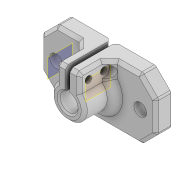
# Autodesk Inventor part: Joint_Mount
Saved by Autodesk Inventor 2020 (Build 240168000, 168)
## iProperties
Created: 2022-01-08
Part Number: Joint_Mount
Material: 一般
Document SubType Name: Modeling
Designer: ken113
Density: 1 g/cm^3
Appearance: 既定
Author: ken113
Autodesk Inventor part; units mm, degrees
ref_plane "YZ Plane" through (0, 0, 0) normal (1, 0, 0) x (0, 1, 0)
ref_plane "XZ Plane" through (0, 0, 0) normal (0, 1, 0) x (-1, 0, 0)
ref_plane "XY Plane" through (0, 0, 0) normal (0, 0, 1) x (1, 0, 0)
sketch "スケッチ1" plane through (0, 0, 0) normal (0, 0, 1) x (1, 0, 0)
  line L0 (37.5, -20) -> (-37.5, -20)
  line L1 (-37.5, -20) -> (-37.5, 20)
  line L2 (-37.5, 20) -> (37.5, 20)
  line L3 (37.5, 20) -> (37.5, -20)
  line L4 (37.5, -20) -> (-37.5, 20) construction
  line L5 (-37.5, -20) -> (37.5, 20) construction
  point P0 (0, 0)
  dimension "d0" = 40
  dimension "d1" = 75
  constraints: 12 end point, 2 midpoint, 2 parallel, 1 horizontal, 1 perpendicular
  measures "d0" distance of L0.end L1.end
  measures "d1" distance of L1.end L2.end
extrude "押し出し1" add sketch "スケッチ1" along normal blind 10
sketch "スケッチ2" plane through (0, 0, 10) normal (0, 0, 1) x (1, 0, 0)
  circle A0 centre (0, 0) radius 5.9
  dimension "d4" = 11.8
  constraints: 1 centre point, 1 coincident
  measures "d4" diameter of A0
extrude "押し出し2" cut sketch "スケッチ2" against normal blind 10
sketch "スケッチ3" plane through (0, 0, 10) normal (0, 0, 1) x (1, 0, 0)
  circle A0 centre (0, 0) radius 5.9
  circle A1 centre (0, 0) radius 10.9
  line L0 (-1.5, 0) -> (1.5, 0)
  line L1 (1.5, 0) -> (1.5, 13.624508)
  line L2 (1.5, 13.624508) -> (-1.5, 13.624508)
  line L3 (-1.5, 13.624508) -> (-1.5, 0)
  point P0 (-1.5, 5.706137)
  point P1 (-1.5, 10.796296)
  point P2 (1.5, 10.796296)
  point P3 (1.5, 5.706137)
  dimension "d7" = 5
  dimension "d8" = 3
  dimension "d9" = 1.5
  constraints: 8 end point, 2 centre point, 2 parallel, 1 coincident, 1 horizontal, 1 perpendicular
  measures "d7" radial gap between concentric circles of A0 A1
  measures "d8" distance of L1.end L2.end
  measures "d9" distance from line of point (0, 0) L3
extrude "押し出し3" add sketch "スケッチ3" along normal blind 20 contours A0 L1 A1 L3 picked at (9.128542, -0.866316)
sketch "スケッチ4" plane through (0, 0, 10) normal (0, 0, 1) x (1, 0, 0)
  line L0 (-1.5, 10.796296) -> (-1.5, 5.706137)
  arc A0 (1.5, 5.706137) -> (-1.5, 5.706137) centre (0, 0) ccw
  line L1 (1.5, 5.706137) -> (1.5, 10.796296)
  arc A1 (-1.5, 10.796296) -> (1.5, 10.796296) centre (0, 0) ccw
  line L2 (-37.5, -20) -> (37.5, -20)
  line L3 (37.5, -20) -> (37.5, 20)
  line L4 (37.5, 20) -> (-37.5, 20)
  line L5 (-37.5, 20) -> (-37.5, -20)
  line L6 (37.5, 20) -> (-37.5, 20)
  line L7 (1.5, 5.706137) -> (-1.5, 5.706137)
  line L8 (-1.5, 5.706137) -> (-1.5, 20)
  line L9 (-1.5, 20) -> (1.5, 20)
  line L10 (1.5, 20) -> (1.5, 5.706137)
  constraints: 8 end point, 2 parallel, 1 horizontal, 1 perpendicular, 1 point on line, 1 vertical alignment
extrude "押し出し4" cut sketch "スケッチ4" against normal blind 20 contours L8 L4 L10 L1 A0 L0
sketch "スケッチ5" plane through (0, 0, 30) normal (0, 0, 1) x (1, 0, 0)
  arc A0 (-1.5, 5.706137) -> (1.5, 5.706137) centre (0, 0) ccw
  line L0 (-1.5, 5.706137) -> (-1.5, 10.796296)
  arc A1 (-1.5, 10.796296) -> (1.5, 10.796296) centre (0, 0) ccw
  line L1 (1.5, 10.796296) -> (1.5, 5.706137)
  line L2 (-1.5, 10.796296) -> (-1.5, 20)
  line L3 (-1.5, 20) -> (-37.5, 20)
  line L4 (-37.5, 20) -> (-37.5, -20)
  line L5 (-37.5, -20) -> (37.5, -20)
  line L6 (37.5, -20) -> (37.5, 20)
  line L7 (37.5, 20) -> (1.5, 20)
  line L8 (1.5, 20) -> (1.5, 10.796296)
  arc A2 (-1.5, 10.796296) -> (1.5, 10.796296) centre (0, 0) ccw
  line L9 (7.5, 1.842007) -> (-7.5, 1.842007)
  line L10 (-7.5, 1.842007) -> (-7.5, 20)
  line L11 (-7.5, 20) -> (7.5, 20)
  line L12 (7.5, 20) -> (7.5, 1.842007)
  point P0 (-1.5, 20)
  point P1 (-7.5, 7.909488)
  point P2 (-1.5, 10.796296)
  point P3 (7.5, 7.909488)
  point P4 (1.5, 20)
  point P5 (1.5, 10.796296)
  dimension "d14" = 6
  dimension "d15" = 6
  constraints: 8 end point, 2 parallel, 1 horizontal, 1 horizontal alignment, 1 perpendicular
  measures "d14" distance between parallel lines of L12 L8
  measures "d15" distance between parallel lines of L10 L2
extrude "押し出し5" add sketch "スケッチ5" against normal up to surface (20 mm away) contours A1 L10 L3 L2 | A1 L8 L7 L12
chamfer "面取り1" distance 5 angle 45 3 edges at (7.5, 13.9547, 10) (0, -10.9, 10) (-7.5, 13.9547, 10)
chamfer "面取り2" distance 2 angle 45 2 edges at (4.5, 20, 30) (-4.5, 20, 30)
chamfer "面取り3" distance 10 angle 45 4 edges at (-37.5, 20, 5) (-37.5, -20, 5) (37.5, 20, 5) (37.5, -20, 5)
chamfer "面取り4" distance 1 angle 45 1 edges at (0, -5.9, 30)
ref_plane "作業平面1" through (12.5, 7.909488, 15) normal (1, 0, 0) x (0, 0, -1)
sketch "スケッチ6" plane through (12.5, 7.909488, 15) normal (1, 0, 0) x (0, 0, -1)
  line L0 (5, 1.917007) -> (5, 12.090512)
  line L1 (5, 12.090512) -> (0, 12.090512)
  line L2 (0, 12.090512) -> (0, 0)
  line L3 (-15, 10.090512) -> (-13, 12.090512)
  line L4 (-15, 0) -> (-15, 10.090512)
  line L5 (0, 0) -> (-15, 0)
  line L6 (0, 12.090512) -> (0, 0)
  line L7 (-13, 12.090512) -> (0, 12.090512)
  point P0 (15, -7.909488)
  point P1 (-9, 6.090512)
  point P2 (1, 6.090512)
  dimension "d32" = 6
  dimension "d33" = 6
  dimension "d34" = 6
  dimension "d35" = 16
  constraints: 1 other
  measures "d32" distance from line of point (-9, 6.091) L7
  measures "d33" distance from line of L7 point (1, 6.091)
  measures "d34" distance from line of point (-9, 6.091) L4
  measures "d35" distance from line of point (1, 6.091) L4
hole "穴1" at (12.5, 14, 24) at (12.5, 14, 14) direction (-1, 0, 0) diameter 4.3 end through all counterbore diameter 8 counterbore depth 5
ref_plane "作業平面2" through (-12.5, 7.909488, 15) normal (-1, 0, 0) x (0, 0, 1)
sketch "スケッチ7" plane through (-12.5, 7.909488, 15) normal (-1, 0, 0) x (0, 0, 1)
  arc A0 (0, 4.187225) -> (0, 7.993799) centre (-1, 6.090512) ccw
  line L0 (0, 0) -> (0, 4.187225)
  line L1 (15, 0) -> (0, 0)
  line L2 (15, 10.090512) -> (15, 0)
  line L3 (13, 12.090512) -> (15, 10.090512)
  line L4 (13, 12.090512) -> (0, 12.090512)
  line L5 (0, 7.993799) -> (0, 12.090512)
  circle A1 centre (9, 6.090512) radius 2.15
  arc A2 (0, 7.993799) -> (0, 4.187225) centre (-1, 6.090512) ccw
  circle A3 centre (9, 6.090512) radius 2.15
  line L6 (4.843078, 6.090512) -> (6.921539, 9.690512)
  line L7 (6.921539, 9.690512) -> (11.078461, 9.690512)
  line L8 (11.078461, 9.690512) -> (13.156922, 6.090512)
  line L9 (13.156922, 6.090512) -> (11.078461, 2.490512)
  line L10 (11.078461, 2.490512) -> (6.921539, 2.490512)
  line L11 (6.921539, 2.490512) -> (4.843078, 6.090512)
  line L12 (3.156922, 6.090512) -> (1.078461, 2.490512)
  line L13 (1.078461, 2.490512) -> (-3.078461, 2.490512)
  line L14 (-3.078461, 2.490512) -> (-5.156922, 6.090512)
  line L15 (-5.156922, 6.090512) -> (-3.078461, 9.690512)
  line L16 (-3.078461, 9.690512) -> (1.078461, 9.690512)
  line L17 (1.078461, 9.690512) -> (3.156922, 6.090512)
  point P0 (-15, -7.909488)
  dimension "d44" = 7.2
  dimension "d45" = 7.2
  constraints: 24 end point, 2 coincident, 1 horizontal alignment, 26 other
  measures "d44" distance between parallel lines of L10 L7
  measures "d45" distance between parallel lines of L13 L16
extrude "押し出し6" cut sketch "スケッチ7" against normal blind 7 contours A0 L5 L16 L17 L12 L13 L0 | L0 L13 L14 L15 L16 L5 A2 | L6 L7 L8 L9 L10 L11
chamfer "面取り5" distance 2 angle 45 2 edges at (1.5, 12.8531, 0) (-1.5, 12.8531, 0)
sketch "スケッチ8" plane through (0, 0, 10) normal (0, 0, 1) x (1, 0, 0)
  line L0 (37.5, -10) -> (27.5, -20)
  line L1 (37.5, -10) -> (37.5, 10)
  line L2 (27.5, 20) -> (37.5, 10)
  line L3 (27.5, 20) -> (12.5, 20)
  line L4 (12.5, 9.826495) -> (12.5, 14)
  arc A0 (-12.5, 9.826495) -> (12.5, 9.826495) centre (0, 0) ccw
  line L5 (-12.5, 20) -> (-12.5, 14.271797)
  line L6 (-12.5, 20) -> (-27.5, 20)
  line L7 (-37.5, 10) -> (-27.5, 20)
  line L8 (-37.5, 10) -> (-37.5, -10)
  line L9 (-27.5, -20) -> (-37.5, -10)
  line L10 (-27.5, -20) -> (27.5, -20)
  line L11 (12.5, 14) -> (12.5, 20)
  line L12 (-12.5, 13.728203) -> (-12.5, 9.826495)
  line L13 (-12.5, 14.271797) -> (-12.5, 13.728203)
  point P0 (27.5, 0)
  point P1 (-27.5, 0)
  dimension "d51" = 10
  dimension "d52" = 10
  measures "d51" distance from line of point (27.5, 0) L1
  measures "d52" distance from line of L8 point (-27.5, 0)
hole "穴2" at (27.5, 0, 10) at (-27.5, 0, 10) direction (0, 0, -1) diameter 8.3 end through all
fillet "フィレット1" radius 2 8 edges at (27.5, -20, 5) (37.5, -10, 5) (37.5, 10, 5) (27.5, 20, 5) (-27.5, 20, 5) (-37.5, 10, 5) (-37.5, -10, 5) (-27.5, -20, 5)
chamfer "面取り6" distance 2 angle 45 26 edges at (-7.5, 12.9547, 30) (-19.5858, 20, 10) (-27.4369, 19.8478, 10) (-32.5, 15, 10) (-37.3478, 9.9369, 10) (-37.5, 0, 10) (-37.3478, -9.9369, 10) (-32.5, -15, 10) (-27.4369, -19.8478, 10) (0, -20, 10) (27.4369, -19.8478, 10) (32.5, -15, 10) (37.3478, -9.9369, 10) (37.5, 0, 10) (37.3478, 9.9369, 10) (32.5, 15, 10) (27.4369, 19.8478, 10) (19.5858, 20, 10) (-10, 20, 12.5) (-7.5, 20, 21.5) (-7.5, 19, 29) (0, -10.9, 30) (7.5, 12.9547, 30) (7.5, 19, 29) (7.5, 20, 21.5) (10, 20, 12.5)
